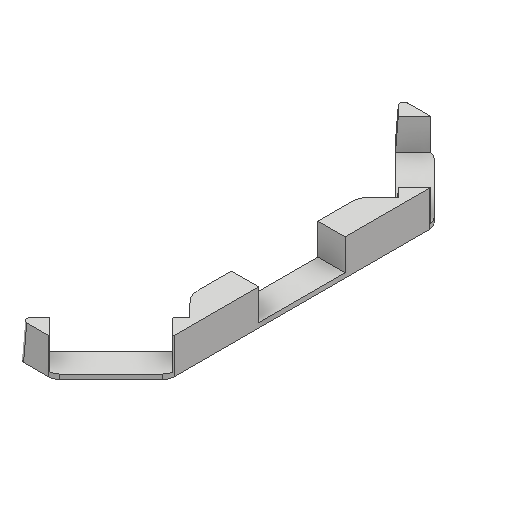
# Autodesk Inventor part: 3DP_PLA_Front_Sharp_sensors_mounting_bracket
Saved by Autodesk Inventor 2025 (Build 290162010, 162A)
## iProperties
Created: 2016-05-23
Part Number: 3DP_PLA_Front_Sharp_sensors_mounting_bracket
Material: Ogólny
Document SubType Name: Modeling
Designer: Andrzej
Density: 1 g/cm^3
Appearance: Domyślna
Author: Andrzej
Autodesk Inventor part; units mm, degrees
ref_plane "YZ Plane" through (0, 0, 0) normal (1, 0, 0) x (0, 1, 0)
ref_plane "XZ Plane" through (0, 0, 0) normal (0, 1, 0) x (-1, 0, 0)
ref_plane "XY Plane" through (0, 0, 0) normal (0, 0, 1) x (1, 0, 0)
sketch "Szkic1" plane through (0, 0, 0) normal (0, 0, 1) x (1, 0, 0)
  arc A0 (-2.9902, -59.8989) -> (-2.4623, -62.135) centre (2.0098, -59.8989) ccw
  line L0 (3.6278, -74.3153) -> (-2.4623, -62.135)
  arc A1 (3.6278, -74.3153) -> (8.1, -77.0792) centre (8.1, -72.0792) ccw
  line L1 (8.1, -77.0792) -> (66.8672, -77.0792)
  arc A2 (66.8672, -77.0792) -> (68.9885, -76.2005) centre (66.8672, -74.0792) ccw
  line L2 (68.9885, -76.2005) -> (82.2311, -62.9579)
  arc A3 (82.2311, -62.9579) -> (83.1098, -60.8366) centre (80.1098, -60.8366) ccw
  line L3 (83.1098, -60.8366) -> (83.1098, 4.6781)
  arc A4 (83.1098, 4.6781) -> (82.2311, 6.7995) centre (80.1098, 4.6781) ccw
  line L4 (82.2311, 6.7995) -> (68.9885, 20.0421)
  arc A5 (68.9885, 20.0421) -> (66.8672, 20.9208) centre (66.8672, 17.9208) ccw
  line L5 (66.8672, 20.9208) -> (8.1, 20.9208)
  arc A6 (8.1, 20.9208) -> (3.6278, 18.1568) centre (8.1, 15.9208) ccw
  line L6 (-2.4623, 5.9765) -> (3.6278, 18.1568)
  arc A7 (-2.4623, 5.9765) -> (-2.9902, 3.7404) centre (2.0098, 3.7404) ccw
  line L7 (-2.9902, 3.7404) -> (-2.9902, -59.8989)
  circle A8 centre (42.0098, -5.5792) radius 1.5
  circle A9 centre (40.0098, -50.5792) radius 1.5
  line L8 (58.8672, 20.9208) -> (58.8672, -77.0792)
  line L9 (76.1098, 3.0213) -> (76.1098, -59.1797)
  line L10 (76.1098, -59.1797) -> (65.2103, -70.0792)
  line L11 (65.2103, 13.9208) -> (76.1098, 3.0213)
  line L12 (65.2103, -70.0792) -> (58.8672, -76.4224)
  line L13 (65.2103, 13.9208) -> (58.8672, 20.2639)
  point P0 (0, 0)
  point P1 (0, 0)
  dimension "d0" = 8
  dimension "d1" = 8
  dimension "d2" = 7
  constraints: 28 end point, 16 point on circle, 10 centre point, 4 point on line, 2 perpendicular, 1 other
  measures "d0" distance from line of L8 L5.start
  measures "d1" distance from line of L8 L1.end
  measures "d2" distance between parallel lines of L3 L9
extrude "Wyciągnięcie proste1" add sketch "Szkic1" along normal blind 9.2 contours L8 L12 L10 L9 L11 L13 L5 A5 L4 A4 L3 A3 L2 A2 L1
sketch "Szkic2" plane through (83.1098, -60.8366, 0) normal (1, 0, 0) x (0, 0, -1)
  line L0 (0, 0) -> (0, 65.5147) projected
  line L1 (0, 65.5147) -> (-9.2, 65.5147) projected
  line L2 (-9.2, 0) -> (-9.2, 65.5147) projected
  line L3 (0, 0) -> (-9.2, 0) projected
  line L4 (-9.2, 21.6324) -> (-1.2, 21.6324)
  line L5 (-1.2, 21.6324) -> (-1.2, 43.8824)
  line L6 (-1.2, 43.8824) -> (-9.2, 43.8824)
  line L7 (-9.2, 43.8824) -> (-9.2, 21.6324)
  point P0 (0, 60.8366)
  dimension "d5" = 8
  dimension "d6" = 22.25
  dimension "d7" = 65.5147
  dimension "d8" = 21.6324
  dimension "d9" = 1.2
  constraints: 8 end point, 2 parallel, 1 horizontal, 1 perpendicular, 1 point on line
  measures "d5" distance of L6.end L5.end
  measures "d6" distance of L5.end L4.end
  measures "d7" distance between parallel lines of L1 L3
  measures "d8" distance between parallel lines of L3 L4
  measures "d9" distance between parallel lines of L0 L5
extrude "Wyciągnięcie proste2" cut sketch "Szkic2" against normal through all contours L2 L6 L5 L4
sketch "Szkic3" plane through (68.9885, 20.0421, 0) normal (0.7071068, 0.7071068, 0) x (-0.7071068, 0.7071068, 0)
  line L0 (-18.7279, 0) -> (0, 0) projected
  line L1 (0, 0) -> (0, 9.2) projected
  line L2 (-18.7279, 9.2) -> (0, 9.2) projected
  line L3 (-18.7279, 0) -> (-18.7279, 9.2) projected
  line L4 (7.3137, 9.2) -> (-17.0711, 9.2) projected
  line L5 (-20.564, 9.2) -> (1.836, 9.2)
  line L6 (1.836, 9.2) -> (1.836, 1.2)
  line L7 (1.836, 1.2) -> (-20.564, 1.2)
  line L8 (-20.564, 1.2) -> (-20.564, 9.2)
  line L9 (-20.8492, 0) -> (-18.7279, 0) projected
  line L10 (-18.7279, 0) -> (-18.7279, 9.2) projected
  line L11 (-20.8492, 9.2) -> (-18.7279, 9.2) projected
  line L12 (-20.8492, 0) -> (-20.8492, 9.2) projected
  line L13 (0, 0) -> (2.1213, 0) projected
  line L14 (2.1213, 0) -> (2.1213, 9.2) projected
  line L15 (0, 9.2) -> (2.1213, 9.2) projected
  line L16 (0, 0) -> (0, 9.2) projected
  point P0 (34.6103, 0)
  dimension "d12" = 22.4
  dimension "d13" = 8
  dimension "d14" = 22.9706
  dimension "d15" = 0.2853
  constraints: 8 end point, 2 parallel, 1 horizontal, 1 perpendicular, 1 point on line
  measures "d12" distance of L6.end L7.end
  measures "d13" distance of L5.end L6.end
  measures "d14" distance between parallel lines of L12 L14
  measures "d15" distance between parallel lines of L12 L8
extrude "Wyciągnięcie proste3" cut sketch "Szkic3" against normal blind 12 contours L7 L8 L5 L3 | L3 L2 L1 L7 | L1 L4 L6 L7
sketch "Szkic4" plane through (82.2311, -62.9579, 9.2) normal (0.7071068, -0.7071068, 0) x (-0.7071068, -0.7071068, 0)
  line L0 (20.8492, 9.2) -> (18.7279, 9.2) projected
  line L1 (18.7279, 9.2) -> (18.7279, 0) projected
  line L2 (20.8492, 0) -> (18.7279, 0) projected
  line L3 (20.8492, 9.2) -> (20.8492, 0) projected
  line L4 (18.7279, 9.2) -> (0, 9.2) projected
  line L5 (0, 9.2) -> (0, 0) projected
  line L6 (18.7279, 0) -> (0, 0) projected
  line L7 (18.7279, 9.2) -> (18.7279, 0) projected
  line L8 (0, 9.2) -> (-2.1213, 9.2) projected
  line L9 (-2.1213, 9.2) -> (-2.1213, 0) projected
  line L10 (0, 0) -> (-2.1213, 0) projected
  line L11 (0, 9.2) -> (0, 0) projected
  line L12 (20.564, 0) -> (-1.836, 0)
  line L13 (-1.836, 0) -> (-1.836, 8)
  line L14 (-1.836, 8) -> (20.564, 8)
  line L15 (20.564, 8) -> (20.564, 0)
  point P0 (13.6282, 9.2)
  dimension "d18" = 22.4
  dimension "d19" = 8
  dimension "d20" = 22.9706
  dimension "d21" = 0.2853
  constraints: 8 end point, 2 parallel, 1 horizontal, 1 perpendicular, 1 point on line
  measures "d18" distance of L13.end L14.end
  measures "d19" distance between parallel lines of L12 L14
  measures "d20" distance between parallel lines of L9 L3
  measures "d21" distance between parallel lines of L3 L15
extrude "Wyciągnięcie proste4" cut sketch "Szkic4" against normal blind 12 contours L14 L15 L2 L1 | L1 L6 L5 L14 | L5 L10 L13 L14
sketch "Szkic5" plane through (83.0857, -61.216, 9.2) normal (-0.7071068, -0.7071068, 0) x (-0.7071068, 0.7071068, 0)
  line L0 (31.2807, 0) -> (31.2807, 8) projected
  line L1 (31.2807, 8) -> (15.5476, 8) projected
  line L2 (15.5476, 8) -> (15.5476, 0) projected
  line L3 (0.2512, 0) -> (15.5476, 0) projected
  line L4 (0.2512, 9.2) -> (0.2512, 0) projected
  line L5 (0.2512, 9.2) -> (46.5771, 9.2) projected
  line L6 (46.5771, 9.2) -> (46.5771, 0) projected
  line L7 (31.2807, 0) -> (46.5771, 0) projected
  line L8 (50.3553, 9.2) -> (6.3725, 9.2) projected
  line L9 (0.2512, 0) -> (15.5476, 0) projected
  line L10 (6.3512, 8) -> (6.3512, 0)
  line L11 (6.3512, 0) -> (10.3512, 0)
  line L12 (10.3512, 0) -> (10.3512, 8)
  line L13 (10.3512, 8) -> (6.3512, 8)
  line L14 (6.3725, 8) -> (9.8654, 8) projected
  point P0 (102.0367, 9.2)
  dimension "d24" = 4
  dimension "d25" = 6.1
  constraints: 8 end point, 2 point on line, 1 parallel
  measures "d24" distance of L11.end L10.end
  measures "d25" distance between parallel lines of L4 L10
extrude "Wyciągnięcie proste5" cut sketch "Szkic5" against normal blind 3.1 contours L3 L10 L13 L12
sketch "Szkic6" plane through (76.1098, -1.9184, 1.2) normal (-0.7071068, 0.7071068, 0) x (-0.7071068, -0.7071068, 0)
  line L0 (5.6822, 8) -> (5.6822, 0) projected
  line L1 (5.6822, 0) -> (21.4153, 0) projected
  line L2 (21.4153, 0) -> (21.4153, 8) projected
  line L3 (36.7117, 8) -> (21.4153, 8) projected
  line L4 (36.7117, -1.2) -> (36.7117, 8) projected
  line L5 (36.7117, -1.2) -> (-9.6142, -1.2) projected
  line L6 (-9.6142, -1.2) -> (-9.6142, 8) projected
  line L7 (5.6822, 8) -> (-9.6142, 8) projected
  line L8 (0, 8) -> (10.6319, 8) projected
  line L9 (5.6822, 0) -> (21.4153, 0) projected
  line L10 (-3.5142, 8) -> (0.4858, 8)
  line L11 (0.4858, 8) -> (0.4858, 0)
  line L12 (0.4858, 0) -> (-3.5142, 0)
  line L13 (-3.5142, 0) -> (-3.5142, 8)
  point P0 (52.4612, -1.2)
  dimension "d28" = 4
  dimension "d29" = 6.1
  constraints: 8 end point, 2 parallel, 2 point on line, 1 horizontal, 1 perpendicular
  measures "d28" distance of L11.end L12.end
  measures "d29" distance between parallel lines of L6 L13
extrude "Wyciągnięcie proste6" cut sketch "Szkic6" against normal blind 3.1 contours L11 L12 L13 L7
fillet "Zaokrąglenie1" radius 5 2 edges at (76.1098, -2.6054, 5.2) (76.1098, -53.553, 5.2)
sketch "Szkic7" plane through (76.1098, -59.1797, 1.2) normal (0, 0, 1) x (1, 0, 0)
  arc A0 (-8.8633, -17.8754) -> (-7.1213, -17.0208) centre (-9.2426, -14.8995) ccw projected
  line L0 (6.1213, -3.7782) -> (-7.1213, -17.0208) projected
  arc A1 (6.1213, -3.7782) -> (6.9759, -2.0362) centre (4, -1.6569) ccw projected
  line L1 (6.9759, -2.0362) -> (2.4849, 2.4548) projected
  line L2 (2.4849, 2.4548) -> (4.677, 4.6468) projected
  line L3 (4.677, 4.6468) -> (1.8485, 7.4752) projected
  arc A2 (0, 11.357) -> (1.8485, 7.4752) centre (5, 11.357) ccw projected
  line L4 (0, 11.357) -> (0, 0) projected
  line L5 (-13.3693, -13.3693) -> (0, 0) projected
  line L6 (-8.8633, -17.8754) -> (-13.3693, -13.3693) projected
  line L7 (0, 50.844) -> (0, 62.201) projected
  arc A3 (1.8485, 54.7258) -> (0, 50.844) centre (5, 50.844) ccw projected
  line L8 (1.8485, 54.7258) -> (4.677, 57.5542) projected
  line L9 (2.4849, 59.7462) -> (4.677, 57.5542) projected
  line L10 (6.9759, 64.2372) -> (2.4849, 59.7462) projected
  arc A4 (6.9759, 64.2372) -> (6.1213, 65.9792) centre (4, 63.8579) ccw projected
  line L11 (-7.1213, 79.2218) -> (6.1213, 65.9792) projected
  arc A5 (-7.1213, 79.2218) -> (-8.8633, 80.0764) centre (-9.2426, 77.1005) ccw projected
  line L12 (-8.8633, 80.0764) -> (-13.3693, 75.5704) projected
  line L13 (0, 62.201) -> (-13.3693, 75.5704) projected
  line L14 (2.4849, 2.4548) -> (4.677, 4.6468) projected
  line L15 (2.4849, 2.4548) -> (0, 0)
  line L16 (2.4849, 59.7462) -> (0, 62.201)
  point P0 (-76.1098, 59.1797)
  constraints: 4 end point
extrude "Wyciągnięcie proste7" cut sketch "Szkic7" against normal through all contours L4 A2 L3 L2 L15 | L7 L16 L9 L8 A3
chamfer "Faza1" distance 0.5 distance2 8 1 edges at (79.6915, -55.6282, 9.2) measured on face at (80.045, -55.9818, 9.2)
chamfer "Faza2" distance 0.5 distance2 8 1 edges at (79.6915, -0.5302, 9.2) measured on face at (80.045, -0.1767, 9.2)
chamfer "Faza3" distance 0.5 distance2 8 1 edges at (60.8038, -74.4857, 9.2) measured on face at (61.1574, -74.8393, 9.2)
chamfer "Faza4" distance 0.5 distance2 8 1 edges at (60.8038, 18.3273, 9.2) measured on face at (61.1574, 18.6808, 9.2)
fillet "Zaokrąglenie4" radius 1 2 edges at (58.8923, 20.9208, 8.9157) (58.8923, -77.0792, 8.9157)
equation "\"d1\" = d0"
equation "\"d8\" = -0.5 * d6 + 0.5 * d7"
equation "\"d15\" = -0.5 * d12 + 0.5 * d14"
equation "\"d21\" = -0.5 * d18 + 0.5 * d20"
